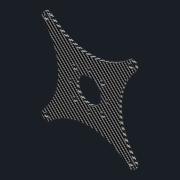
# Autodesk Inventor part: unit-j2-plate2
Saved by Autodesk Inventor 2021 (Build 250183000, 183)
## iProperties
Created: 2021-07-12
Part Number: unit-j2-plate2
Material: CFRP
Document SubType Name: Sheet Metal
Designer: yuta0
Density: 1.43 g/cm^3
Sheet Metal Rule: Default_mm
Appearance: カーボンファイバー
Mass: 23.7815 g
Surface Area: 177.903 cm^2
Volume: 16.6304 cm^3
購入先: カーボン
在庫数: 0.0
Author: yuta0
Autodesk Inventor part; units mm, degrees
ref_plane "YZ Plane" through (0, 0, 0) normal (1, 0, 0) x (0, 1, 0)
ref_plane "XZ Plane" through (0, 0, 0) normal (0, 1, 0) x (-1, 0, 0)
ref_plane "XY Plane" through (0, 0, 0) normal (0, 0, 1) x (1, 0, 0)
sketch "スケッチ1" plane through (0, 0, 0) normal (0, 0, 1) x (1, 0, 0)
  circle A0 centre (0, 0) radius 75
  dimension "d0" = 150
  measures "d0" diameter of A0
extrude "プレート1" add sketch "スケッチ1" along normal blind 2
sketch "スケッチ2" plane through (0, 0, 2) normal (0, 0, 1) x (1, 0, 0)
  circle A0 centre (0, 0) radius 10
  dimension "d2" = 20
  constraints: 1 centre point, 1 coincident
  measures "d2" diameter of A0
extrude "押し出し1" cut sketch "スケッチ2" against normal through all
sketch "スケッチ4" plane through (0, 0, 2) normal (0, 0, 1) x (1, 0, 0)
  circle A0 centre (0, 0) radius 49
  point P0 (34.6482, 34.6482)
  point P1 (-34.6482, 34.6482)
  point P2 (-34.6482, -34.6482)
  point P3 (34.6482, -34.6482)
  dimension "d17" = 98
  dimension "d20" = 360
  dimension "d55" = 0
  constraints: 1 coincident, 8 other
  measures "d55" vertical distance of point (-34.648, 34.648) point (34.648, 34.648)
hole "穴2" at (34.6482, 34.6482, 2) at (-34.6482, 34.6482, 2) at (-34.6482, -34.6482, 2) at (34.6482, -34.6482, 2) direction (0, 0, -1) diameter 4.3 end through all clearance for "Flat Head Machine Screw" size "M4" standard "Ansi Metric M Profile"
sketch "スケッチ5" plane through (0, 0, 0) normal (0, 0, -1) x (-1, 0, 0)
  circle A0 centre (0, 0) radius 16
  point P0 (11.3137, 11.3137)
  point P1 (-11.3137, 11.3137)
  point P2 (-11.3137, -11.3137)
  point P3 (11.3137, -11.3137)
  dimension "d29" = 32
  dimension "d32" = 360
  constraints: 1 coincident, 1 vertical alignment, 8 other
hole "穴3" at (-11.3137, 11.3137, 0) at (11.3137, 11.3137, 0) at (11.3137, -11.3137, 0) at (-11.3137, -11.3137, 0) direction (0, 0, 1) diameter 4.3 depth 2 tip angle 118 clearance for "Flat Head Machine Screw" size "M4" standard "Ansi Metric M Profile"
sketch "スケッチ6" plane through (0, 0, 0) normal (0, 0, -1) x (-1, 0, 0)
  circle A0 centre (0, 0) radius 15
  point P0 (0, 15)
  point P1 (-15, 0)
  point P2 (0, -15)
  point P3 (15, 0)
  dimension "d41" = 30
  dimension "d44" = 360
  constraints: 2 vertical alignment, 1 coincident, 7 other
hole "穴4" at (0, 15, 0) at (15, 0, 0) at (0, -15, 0) at (-15, 0, 0) direction (0, 0, 1) diameter 3.2 depth 2 tip angle 118 clearance for "Flat Head Machine Screw" size "M3" standard "Ansi Metric M Profile"
sketch "スケッチ8" plane through (0, 0, 0) normal (0, 0, -1) x (-1, 0, 0)
  circle A0 centre (-34.6482, 34.6482) radius 2.15 projected
  line L0 (34.6482, -34.6482) -> (-34.6482, -34.6482)
  line L1 (-34.6482, -34.6482) -> (-34.6482, 34.6482)
  line L2 (-34.6482, 34.6482) -> (34.6482, 34.6482)
  line L3 (34.6482, 34.6482) -> (34.6482, -34.6482)
  line L4 (34.6482, -34.6482) -> (-34.6482, 34.6482) construction
  line L5 (-34.6482, -34.6482) -> (34.6482, 34.6482) construction
  line L6 (38.6482, -38.6482) -> (-38.6482, -38.6482)
  line L7 (-38.6482, -38.6482) -> (-38.6482, 38.6482)
  line L8 (-38.6482, 38.6482) -> (38.6482, 38.6482)
  line L9 (38.6482, 38.6482) -> (38.6482, -38.6482)
  line L10 (38.6482, -38.6482) -> (-38.6482, 38.6482) construction
  line L11 (-38.6482, -38.6482) -> (38.6482, 38.6482) construction
  circle A1 centre (0, 0) radius 75 projected
  dimension "d56" = 4
  constraints: 24 end point, 4 midpoint, 4 parallel, 2 horizontal, 2 perpendicular, 1 point on line
  measures "d56" distance between parallel lines of L8 L2
extrude "押し出し2" cut sketch "スケッチ8" against normal blind 10 contours A1
fillet "コーナーR1" radius 4 4 edges at (38.6482, 38.6482, 1) (-38.6482, 38.6482, 1) (-38.6482, -38.6482, 1) (38.6482, -38.6482, 1)
sketch "スケッチ9" plane through (0, 0, 2) normal (0, 0, 1) x (1, 0, 0)
  circle A0 centre (-34.6482, 34.6482) radius 2.15 projected
  circle A1 centre (34.6482, 34.6482) radius 2.15 projected
  circle A2 centre (34.6482, -34.6482) radius 2.15 projected
  circle A3 centre (-34.6482, -34.6482) radius 2.15 projected
  circle A4 centre (-34.6482, 34.6482) radius 4
  circle A5 centre (34.6482, 34.6482) radius 4
  circle A6 centre (0, 71.8042) radius 46.8042
  line L0 (34.6482, 38.6482) -> (-34.6482, 38.6482) projected
  line L1 (-38.6482, 34.6482) -> (-38.6482, -34.6482) projected
  line L2 (38.6482, -34.6482) -> (38.6482, 34.6482) projected
  line L3 (-34.6482, -38.6482) -> (34.6482, -38.6482) projected
  point P0 (0, 0)
  point P1 (0, 25)
  point P2 (-31.9202, 37.5737)
  point P3 (31.9202, 37.5737)
  dimension "d60" = 8
  dimension "d61" = 8
  dimension "d62" = 25
  constraints: 2 centre point, 2 coincident, 5 other
  measures "d60" diameter of A4
  measures "d61" diameter of A5
  measures "d62" distance of point (0, 0) point (0, 25)
extrude "押し出し3" cut sketch "スケッチ9" against normal blind 10 contours L0 A6 A4 | A6 L0 | A6 L0 A5 picked at (8.3251, 35.7892)
pattern_circular "円形状パターン1" count 4 over 360 about axis through (0, 0, -10) along (0, 0, 1) of "押し出し3"
equation "\"d27\" = Thickness"
equation "\"d39\" = Thickness"
equation "\"d51\" = Thickness"
equation "\"d1\" = Thickness"
equation "\"BendRadius\" = Thickness"
equation "\"BendReliefWidth\" = Thickness"
equation "\"BendReliefDepth\" = 0.5 * Thickness"
equation "\"CornerReliefSize\" = 4 * Thickness"
equation "\"MinimumRemnant\" = 2 * Thickness"
equation "\"TransitionRadius\" = BendRadius"
equation "\"JacobiRadiusSize\" = BendRadius"
equation "\"GapSize\" = Thickness"
equation "\"Thickness\" = 2"
